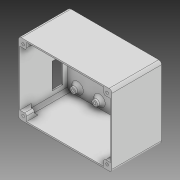
# Autodesk Inventor part: MainEnclosure
Saved by Autodesk Inventor 2020 (Build 240168000, 168)
## iProperties
Created: 2021-01-12
Part Number: MainEnclosure
Material: Generic
Document SubType Name: Modeling
Designer: DDeGo
Density: 1 g/cm^3
Appearance: Default
Author: DDeGo
Autodesk Inventor part; units mm, degrees
ref_plane "YZ Plane" through (0, 0, 0) normal (1, 0, 0) x (0, 1, 0)
ref_plane "XZ Plane" through (0, 0, 0) normal (0, 1, 0) x (-1, 0, 0)
ref_plane "XY Plane" through (0, 0, 0) normal (0, 0, 1) x (1, 0, 0)
sketch "Sketch1" plane through (0, 0, 0) normal (0, 0, 1) x (1, 0, 0)
  line L0 (-47.5, -36) -> (47.5, -36) construction
  line L1 (47.5, -36) -> (47.5, 36) construction
  line L2 (47.5, 36) -> (-47.5, 36) construction
  line L3 (-47.5, 36) -> (-47.5, -36) construction
  line L4 (-47.5, -36) -> (47.5, 36) construction
  line L5 (47.5, -36) -> (-47.5, 36) construction
  line L6 (49, -37.5) -> (-49, -37.5)
  line L7 (-49, -37.5) -> (-49, 37.5)
  line L8 (-49, 37.5) -> (49, 37.5)
  line L9 (49, 37.5) -> (49, -37.5)
  line L10 (49, -37.5) -> (-49, 37.5) construction
  line L11 (-49, -37.5) -> (49, 37.5) construction
  point P0 (0, 0)
  dimension "d0" = 72
  dimension "d1" = 95
  dimension "d2" = 1.5
  dimension "d3" = 1.5
  constraints: 24 end point, 4 midpoint, 4 parallel, 2 horizontal, 2 perpendicular
  measures "d0" distance of L2.end L0.start
  measures "d1" distance of L1.end L2.end
  measures "d2" distance between parallel lines of L8 L2
  measures "d3" distance between parallel lines of L7 L3
extrude "Extrusion1" add sketch "Sketch1" along normal blind 2
sketch "Sketch2" plane through (0, 0, 2) normal (0, 0, 1) x (1, 0, 0)
  line L0 (47.5, -36) -> (-47.5, -36)
  line L1 (-47.5, -36) -> (-47.5, 36)
  line L2 (-47.5, 36) -> (47.5, 36)
  line L3 (47.5, 36) -> (47.5, -36)
  line L4 (47.5, -36) -> (-47.5, 36) construction
  line L5 (-47.5, -36) -> (47.5, 36) construction
  line L6 (49, 37.5) -> (-49, 37.5) projected
  line L7 (-49, 37.5) -> (-49, -37.5) projected
  line L8 (-49, -37.5) -> (49, -37.5) projected
  line L9 (49, -37.5) -> (49, 37.5) projected
  point P0 (0, 0)
  constraints: 12 end point, 2 midpoint, 2 parallel, 1 coincident, 1 horizontal, 1 perpendicular
extrude "Extrusion2" add sketch "Sketch2" along normal blind 50
sketch "Sketch3" plane through (0, 0, 0) normal (0, 1, 0) x (-1, 0, 0)
  line L0 (-47.5, 2) -> (47.5, 2) projected
  line L1 (49, 0) -> (-49, 0) projected
  line L2 (-47.5, 2) -> (-47.5, 52) projected
  line L3 (-19, 0) -> (-48, 0)
  line L4 (-48, 0) -> (-46, 2)
  line L5 (-46, 2) -> (-19, 2)
  line L6 (-19, 0) -> (-19, 2)
  line L7 (-49, 0) -> (-49, 52) projected
  point P0 (0, 0)
  dimension "d8" = 45
  dimension "d9" = 29
  dimension "d10" = 1
  constraints: 8 end point, 4 point on line, 1 perpendicular
  measures "d8" angle of L1 L4
  measures "d9" distance of L3.end L3.start
  measures "d10" distance from line of L3.end L7
revolve "Revolution1" cut sketch "Sketch3" angle 360 about axis through (19, 0, 0) along (0, 0, 1)
sketch "Sketch4" plane through (0, 0, 0) normal (0, 1, 0) x (-1, 0, 0)
  line L0 (-46, 2) -> (8, 2) projected
  line L1 (-46, 2) -> (-44.5, 3.5)
  line L2 (-44.5, 3.5) -> (-46.5, 3.5)
  line L3 (-46.5, 3.5) -> (-48, 2)
  line L4 (-48, 2) -> (-46, 2)
  line L5 (10, 0) -> (-48, 0) projected
  line L6 (-48, 0) -> (-46, 2) projected
  line L7 (-19, 0) -> (-19, 2) projected
  point P0 (0, 0)
  dimension "d12" = 2
  dimension "d13" = 1.5
  constraints: 8 end point, 2 parallel, 1 collinear, 1 horizontal
  measures "d12" distance of L3.end L1.start
  measures "d13" distance between parallel lines of L4 L2
revolve "Revolution2" add sketch "Sketch4" angle 360 about axis through (19, 0, 0) along (0, 0, 1) contours L4 L3 L2 L1
fillet "Fillet1" radius 3 1 edges at (-10, 0, 2)
sketch "Sketch5" plane through (0, 0, 2) normal (0, 0, 1) x (1, 0, 0)
  line L0 (-47.5, 36) -> (47.5, 36) projected
  line L1 (-47.5, -36) -> (-47.5, 36) projected
  line L2 (-40.5, -32) -> (-40.5, 33) construction
  line L3 (-40.5, 33) -> (-10.5, 33) construction
  line L4 (-10.5, 33) -> (-10.5, -32) construction
  line L5 (-10.5, -32) -> (-40.5, -32) construction
  line L6 (-40.5, -32) -> (-10.5, 33) construction
  line L7 (-40.5, 33) -> (-10.5, -32) construction
  line L8 (-37, -28.5) -> (-37, 29.5) construction
  line L9 (-37, 29.5) -> (-14, 29.5) construction
  line L10 (-14, 29.5) -> (-14, -28.5) construction
  line L11 (-14, -28.5) -> (-37, -28.5) construction
  line L12 (-37, -28.5) -> (-14, 29.5) construction
  line L13 (-37, 29.5) -> (-14, -28.5) construction
  circle A0 centre (-37, 29.5) radius 3
  circle A1 centre (-14, 29.5) radius 3
  circle A2 centre (-14, -28.5) radius 3
  circle A3 centre (-37, -28.5) radius 3
  circle A4 centre (-37, -28.5) radius 1.35
  circle A5 centre (-37, 29.5) radius 1.35
  circle A6 centre (-14, 29.5) radius 1.35
  circle A7 centre (-14, -28.5) radius 1.35
  point P0 (-12.8395, 36.7828)
  dimension "d25" = 3
  dimension "d26" = 7
extrude "Extrusion3" add sketch "Sketch5" along normal blind 5
fillet "Fillet2" radius 3 4 edges at (-40, 29.5, 2) (-17, 29.5, 2) (-17, -28.5, 2) (-40, -28.5, 2)
sketch "Sketch6" plane through (-49, -37.5, 0) normal (-1, 0, 0) x (0, 0, 1)
  line L0 (7, 10.35) -> (7, 7.65) construction
  line L1 (7, 9) -> (18, 9)
  line L2 (18, 9) -> (18, 36)
  line L3 (18, 36) -> (7, 36)
  line L4 (7, 36) -> (7, 9)
  point P0 (0, 37.5)
  dimension "d30" = 11
  dimension "d31" = 27
  constraints: 8 end point, 2 parallel, 1 horizontal, 1 midpoint, 1 perpendicular
  measures "d30" distance of L1.start L1.end
  measures "d31" distance of L3.end L1.start
extrude "Extrusion4" cut sketch "Sketch6" against normal up to surface (1.5 mm away)
sketch "Sketch7" plane through (0, 0, 52) normal (0, 0, 1) x (1, 0, 0)
  line L0 (0, 0) -> (29.4797, 0) construction
  line L1 (-47.5, -36) -> (-47.5, 36) projected
  line L2 (-42.5, 29) -> (-47.5, 29)
  line L3 (-47.5, 29) -> (-47.5, 36)
  line L4 (-47.5, 36) -> (-40.5, 36)
  line L5 (-40.5, 36) -> (-40.5, 31)
  line L6 (-40.5, 29) -> (-47.5, 36) construction
  line L7 (-47.5, 29) -> (-40.5, 36) construction
  line L8 (47.5, 36) -> (-47.5, 36) projected
  line L9 (42.5, 29) -> (47.5, 29)
  line L10 (47.5, 29) -> (47.5, 36)
  line L11 (47.5, 36) -> (40.5, 36)
  line L12 (40.5, 36) -> (40.5, 31)
  line L13 (40.5, 29) -> (47.5, 36) construction
  line L14 (47.5, 29) -> (40.5, 36) construction
  circle A0 centre (-44, 32.5) radius 1.4
  circle A1 centre (44, 32.5) radius 1.4
  arc A2 (-42.5, 29) -> (-40.5, 31) centre (-42.5, 31) ccw
  arc A3 (40.5, 31) -> (42.5, 29) centre (42.5, 31) ccw
  line L15 (-42.5, -29) -> (-47.5, -29)
  line L16 (-47.5, -29) -> (-47.5, -36)
  line L17 (-47.5, -36) -> (-40.5, -36)
  line L18 (-40.5, -36) -> (-40.5, -31)
  line L19 (-40.5, -29) -> (-47.5, -36) construction
  line L20 (-47.5, -29) -> (-40.5, -36) construction
  line L21 (-47.5, -36) -> (47.5, -36) projected
  line L22 (42.5, -29) -> (47.5, -29)
  line L23 (47.5, -29) -> (47.5, -36)
  line L24 (47.5, -36) -> (40.5, -36)
  line L25 (40.5, -36) -> (40.5, -31)
  line L26 (40.5, -29) -> (47.5, -36) construction
  line L27 (47.5, -29) -> (40.5, -36) construction
  arc A4 (-40.5, -31) -> (-42.5, -29) centre (-42.5, -31) ccw
  arc A5 (42.5, -29) -> (40.5, -31) centre (42.5, -31) ccw
  circle A6 centre (-44, -32.5) radius 1.4
  circle A7 centre (44, -32.5) radius 1.4
  point P0 (44, -32.5)
  dimension "d34" = 7
  dimension "d35" = 2.8
  dimension "d36" = 2
  dimension "d37" = 2
  constraints: 50 end point, 8 centre point, 8 midpoint, 8 parallel, 8 point on circle, 8 point on line, 8 tangent, 7 equal length, 5 equal radius, 5 horizontal, 4 coincident, 4 perpendicular
  measures "d34" distance of L4.end L6.start
  measures "d35" diameter of A0
  measures "d36" radius of A2
  measures "d37" radius of A4
extrude "Extrusion5" add sketch "Sketch7" against normal blind 8
chamfer "Chamfer1" distance 4 angle 45 8 edges at (-47.5, 32.5, 44) (-44, 36, 44) (47.5, 32.5, 44) (44, 36, 44) (47.5, -32.5, 44) (44, -36, 44) (-47.5, -32.5, 44) (-44, -36, 44)
fillet "Fillet3" radius 3 8 edges at (47.5, -36, 21) (-49, -37.5, 26) (-47.5, -36, 21) (-49, 37.5, 26) (47.5, 36, 21) (49, 37.5, 26) (49, -37.5, 26) (-47.5, 36, 21)
sketch "Block2" plane through (0, 0, 0) normal (0, 0, 1) x (1, 0, 0)
  line L0 (113, 2) -> (48, 2) construction
  line L1 (48, 2) -> (48, 32) construction
  line L2 (48, 32) -> (113, 32) construction
  line L3 (113, 32) -> (113, 2) construction
  line L4 (113, 2) -> (48, 32) construction
  line L5 (48, 2) -> (113, 32) construction
  line L6 (109.5, 5.5) -> (51.5, 5.5) construction
  line L7 (51.5, 5.5) -> (51.5, 28.5) construction
  line L8 (51.5, 28.5) -> (109.5, 28.5) construction
  line L9 (109.5, 28.5) -> (109.5, 5.5) construction
  line L10 (109.5, 5.5) -> (51.5, 28.5) construction
  line L11 (51.5, 5.5) -> (109.5, 28.5) construction
  circle A0 centre (51.5, 5.5) radius 3
  circle A1 centre (51.5, 28.5) radius 3
  circle A2 centre (109.5, 28.5) radius 3
  circle A3 centre (109.5, 5.5) radius 3
  circle A4 centre (109.5, 5.5) radius 1.35
  circle A5 centre (51.5, 5.5) radius 1.35
  circle A6 centre (51.5, 28.5) radius 1.35
  circle A7 centre (109.5, 28.5) radius 1.35
  point P0 (80.5, 17)
  point P1 (80.5, 17)
  point P2 (80.5, 17)
  dimension "d16" = 23
  dimension "d17" = 58
  dimension "d18" = 30
  dimension "d19" = 65
  dimension "d20" = 2.7
  dimension "d21" = 6
  constraints: 24 end point, 8 centre point, 8 coincident, 6 equal radius, 5 midpoint, 4 parallel, 2 horizontal, 2 perpendicular
  measures "d16" distance of L6.end L7.end
  measures "d17" distance of L7.end L8.end
  measures "d18" distance of L0.end L1.end
  measures "d19" distance of L1.end L2.end
  measures "d20" diameter of A5
  measures "d21" diameter of A0
body "Solid1"
